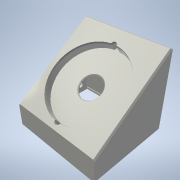
# Autodesk Inventor part: BARB_top
Saved by Autodesk Inventor 2022.3 (Build 263350000, 350)
## iProperties
Created: 2022-06-21
Part Number: BARB_top
Material: ABS Plastic
Document SubType Name: Modeling
Designer: abmos
Density: 1.06 g/cm^3
Appearance: Smooth - Ivory
Author: abmos
Autodesk Inventor part; units mm, degrees
ref_plane "YZ Plane" through (0, 0, 0) normal (1, 0, 0) x (0, 1, 0)
ref_plane "XZ Plane" through (0, 0, 0) normal (0, 1, 0) x (-1, 0, 0)
sketch "XZ_master" plane through (0, 0, 0) normal (0, 1, 0) x (-1, 0, 0)
  line L0 (52.5, -47.5) -> (-52.5, -47.5)
  line L1 (-52.5, -47.5) -> (-52.5, 47.5)
  line L2 (-52.5, 47.5) -> (52.5, 47.5)
  line L3 (52.5, 47.5) -> (52.5, -47.5)
  line L4 (52.5, -47.5) -> (-52.5, 47.5) construction
  line L5 (-52.5, -47.5) -> (52.5, 47.5) construction
  line L6 (50.5, -45.5) -> (-50.5, -45.5)
  line L7 (-50.5, -45.5) -> (-50.5, 45.5)
  line L8 (-50.5, 45.5) -> (50.5, 45.5)
  line L9 (50.5, 45.5) -> (50.5, -45.5)
  point P0 (0, 0)
  dimension "d0" = 105
  dimension "d1" = 95
  dimension "d2" = 2
  constraints: 20 end point, 4 parallel, 2 midpoint, 2 perpendicular, 1 horizontal, 3 other
  measures "d0" distance of L1.end L2.end
  measures "d1" distance of L0.end L1.end
  measures "d2" distance between parallel lines of L3 L9
sketch "XZ_master outline for Walls_bottom" plane through (0, 0, 0) normal (0, 1, 0) x (-1, 0, 0)
  line L0 (52.5, -47.5) -> (52.5, 47.5)
  line L1 (-52.5, -47.5) -> (52.5, -47.5)
  line L2 (52.5, 47.5) -> (-52.5, 47.5)
  line L3 (-52.5, 47.5) -> (-52.5, -47.5)
  line L4 (50.5, -45.5) -> (-50.5, -45.5)
  line L5 (50.5, 45.5) -> (50.5, -45.5)
  line L6 (-50.5, 45.5) -> (50.5, 45.5)
  line L7 (-50.5, -45.5) -> (-50.5, 45.5)
extrude "Walls_bottom" add sketch "XZ_master outline for Walls_bottom" along normal blind 25
fillet "Fillet2" radius 0.75 4 edges at (0, 0, 45.5) (50.5, 0, 0) (-50.5, 0, 0) (0, 0, -45.5)
sketch "Profile" plane through (0, 0, 0) normal (1, 0, 0) x (0, 1, 0)
  line L0 (0, 45.5) -> (25, 45.5)
  line L1 (2, 45.5) -> (4, 45.5)
  line L2 (4, 45.5) -> (4, 46.7)
  line L3 (4, 46.7) -> (2, 46.7)
  line L4 (2, 46.7) -> (2, 45.5)
  line L5 (0, -47.5) -> (0, 47.5)
  circle A0 centre (10.654636, -35.042492) radius 3.75
  line L6 (4, 46.7) -> (4, -38.2) construction
  line L7 (4, 46.7) -> (88.9, 46.7) construction
  point P0 (0, 0)
  dimension "d5" = 2
  dimension "d6" = 1.2
  dimension "d7" = 2
  dimension "d27" = 7.5
  dimension "d30" = 90
  constraints: 12 end point, 2 horizontal, 2 parallel, 2 perpendicular, 1 centre point, 1 point on line
  measures "d5" distance of L3.end L2.end
  measures "d6" distance of L2.end L1.end
  measures "d7" distance between parallel lines of L5 L4
  measures "d27" diameter of A0
  measures "d30" angle of L6 L7
sketch "Profile outline for Lip recess" plane through (0, 0, 0) normal (1, 0, 0) x (0, 1, 0)
  line L0 (4, 46.7) -> (2, 46.7)
  line L1 (4, 45.5) -> (4, 46.7)
  line L2 (2, 45.5) -> (4, 45.5)
  line L3 (2, 46.7) -> (2, 45.5)
extrude "Lip recess" cut sketch "Profile outline for Lip recess" along normal mid plane 101
fillet "Lip_fillet" radius 1 2 edges at (0, 4, 45.5) (0, 2, 45.5)
pattern_circular "Circular Pattern1" count 2 over 360 about axis through (0, -10, 0) along (0, 1, 0) of "Lip recess"
ref_plane "Angled_top_face" through (-52.5, 25, 47.5) normal (0, -0.819152, -0.5735764) x (1, 0, 0)
sketch "XZ_master outline for Walls_to_workplane" plane through (0, 0, 0) normal (0, 1, 0) x (-1, 0, 0)
  line L0 (52.5, -47.5) -> (52.5, 47.5)
  line L1 (-52.5, -47.5) -> (52.5, -47.5)
  line L2 (52.5, 47.5) -> (-52.5, 47.5)
  line L3 (-52.5, 47.5) -> (-52.5, -47.5)
  line L4 (50.5, -45.5) -> (-50.5, -45.5)
  line L5 (50.5, 45.5) -> (50.5, -45.5)
  line L6 (-50.5, 45.5) -> (50.5, 45.5)
  line L7 (-50.5, -45.5) -> (-50.5, 45.5)
extrude "Walls_to_workplane" add sketch "XZ_master outline for Walls_to_workplane" along normal up to surface from surface at 25 surface through (-52.5, 25, 47.5) normal (0, -0.819152, -0.5735764)
sketch "Top_face" plane through (-52.5, 25, 47.5) normal (0, -0.819152, -0.5735764) x (1, 0, 0)
  line L0 (105, -115.973586) -> (0, -115.973586)
  line L1 (0, 0) -> (105, 0)
  line L2 (105, 0) -> (105, -115.973586)
  line L3 (105, -115.973586) -> (0, -115.973586)
  line L4 (0, -115.973586) -> (0, 0)
  line L5 (0, -115.973586) -> (0, 0) construction
  line L6 (2, -2.441549) -> (2, -113.532037)
  line L7 (2, -113.532037) -> (103, -113.532037)
  line L8 (103, -113.532037) -> (103, -2.441549)
  line L9 (103, -2.441549) -> (2, -2.441549)
  line L10 (105, 0) -> (105, -115.973586)
  line L11 (105, -115.973586) -> (0, -115.973586)
  line L12 (0, -115.973586) -> (0, 0)
  line L13 (0, 0) -> (105, 0)
  line L14 (2, -113.532037) -> (103, -113.532037) construction
  line L15 (52.5, -113.532037) -> (52.5, -2.441549) construction
  line L16 (103, -2.441549) -> (2, -2.441549) construction
  circle A0 centre (52.5, -53.441549) radius 44
  circle A1 centre (52.5, -97.441549) radius 3
  circle A2 centre (52.5, -9.441549) radius 3
  circle A3 centre (52.5, -53.441549) radius 46
  circle A4 centre (52.5, -97.441549) radius 5
  circle A5 centre (52.5, -9.441549) radius 5
  circle A6 centre (52.5, -53.441549) radius 13.5
  circle A7 centre (52.5, -53.441549) radius 51 construction
  point P0 (55.498256, -97.339276)
  point P1 (55.498256, -9.543822)
  point P2 (49.501744, -9.543822)
  point P3 (49.501744, -97.339276)
  point P4 (47.820513, -99.202913)
  point P5 (57.179487, -99.202913)
  point P6 (57.179487, -7.680186)
  point P7 (47.820513, -7.680186)
  dimension "d61" = 88
  dimension "d62" = 51
  dimension "d63" = 6
  dimension "d64" = 6
  dimension "d65" = 2
  dimension "d66" = 2
  dimension "d67" = 2
  dimension "d68" = 27
  dimension "d69" = 102
  constraints: 10 end point, 8 centre point, 3 point on line, 2 coincident, 2 midpoint, 2 parallel, 2 point on circle, 1 horizontal, 1 perpendicular
  measures "d61" diameter of A0
  measures "d62" distance from line of L9 A3.centre
  measures "d63" diameter of A1
  measures "d64" diameter of A2
  measures "d65" radial gap between concentric circles of A0 A3
  measures "d66" radial gap between concentric circles of A1 A4
  measures "d67" radial gap between concentric circles of A2 A5
  measures "d68" diameter of A6
  measures "d69" diameter of A7
sketch "Top_face outline for Face" plane through (-52.5, 25, 47.5) normal (0, -0.819152, -0.5735764) x (1, 0, 0)
  line L0 (105, -115.973586) -> (105, 0)
  line L1 (0, -115.973586) -> (105, -115.973586)
  line L2 (0, 0) -> (0, -115.973586)
  line L3 (105, 0) -> (0, 0)
extrude "Face" add sketch "Top_face outline for Face" against normal blind 2 draft -35
sketch "Top_face outline for Button_recess" plane through (-52.5, 25, 47.5) normal (0, -0.819152, -0.5735764) x (1, 0, 0)
  arc A0 (49.501744, -97.339276) -> (55.498256, -97.339276) centre (52.5, -97.441549) ccw
  arc A1 (49.501744, -9.543822) -> (49.501744, -97.339276) centre (52.5, -53.441549) ccw
  arc A2 (55.498256, -9.543822) -> (49.501744, -9.543822) centre (52.5, -9.441549) ccw
  arc A3 (55.498256, -97.339276) -> (55.498256, -9.543822) centre (52.5, -53.441549) ccw
extrude "Button_recess" cut sketch "Top_face outline for Button_recess" against normal through all draft 15
sketch "Profile outline for Side_cable_cutout" plane through (0, 0, 0) normal (1, 0, 0) x (0, 1, 0)
  circle A0 centre (10.654636, -35.042492) radius 3.75
extrude "Side_cable_cutout" cut sketch "Profile outline for Side_cable_cutout" against normal through all
sketch "Top_face outline for Recess_walls" plane through (-52.5, 25, 47.5) normal (0, -0.819152, -0.5735764) x (1, 0, 0)
  arc A0 (47.820513, -99.202913) -> (57.179487, -99.202913) centre (52.5, -97.441549) ccw
  arc A1 (47.820513, -7.680186) -> (47.820513, -99.202913) centre (52.5, -53.441549) ccw
  arc A2 (57.179487, -99.202913) -> (57.179487, -7.680186) centre (52.5, -53.441549) ccw
  arc A3 (57.179487, -7.680186) -> (47.820513, -7.680186) centre (52.5, -9.441549) ccw
  arc A4 (55.498256, -97.339276) -> (49.501744, -97.339276) centre (52.5, -97.441549) cw
  arc A5 (55.498256, -9.543822) -> (55.498256, -97.339276) centre (52.5, -53.441549) cw
  arc A6 (49.501744, -9.543822) -> (55.498256, -9.543822) centre (52.5, -9.441549) cw
  arc A7 (49.501744, -97.339276) -> (49.501744, -9.543822) centre (52.5, -53.441549) cw
extrude "Recess_walls" add sketch "Top_face outline for Recess_walls" along normal blind 8.5
sketch "Top_face outline for Recess_floor" plane through (-52.5, 25, 47.5) normal (0, -0.819152, -0.5735764) x (1, 0, 0)
  arc A0 (47.820513, -99.202913) -> (57.179487, -99.202913) centre (52.5, -97.441549) ccw
  arc A1 (47.820513, -7.680186) -> (47.820513, -99.202913) centre (52.5, -53.441549) ccw
  arc A2 (57.179487, -99.202913) -> (57.179487, -7.680186) centre (52.5, -53.441549) ccw
  arc A3 (57.179487, -7.680186) -> (47.820513, -7.680186) centre (52.5, -9.441549) ccw
  circle A4 centre (52.5, -53.441549) radius 13.5
extrude "Recess_floor" add sketch "Top_face outline for Recess_floor" along normal blind 2 from surface at 8.5
chamfer "Button_cutout_chamfer" distance 1 angle 45 1 edges at (-13.5, 48.69, -1.1522)
body "Solid1"
